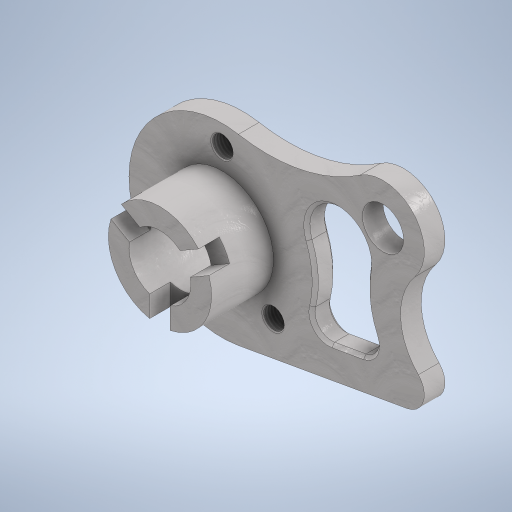
# Autodesk Inventor part: Curved Disc new
Saved by Autodesk Inventor 2023 (Build 270158030, 158C)
## iProperties
Created: 2020-06-23
Part Number: Curved Disc new
Material: Steel, Mild, Welded
Document SubType Name: Modeling
Designer: Smit Ambardekar
Density: 7.85 g/cm^3
Appearance: Weld - Steel Mild
Author: Smit Ambardekar
Autodesk Inventor part; units mm, degrees
ref_plane "YZ Plane" through (0, 0, 0) normal (1, 0, 0) x (0, 1, 0)
ref_plane "XZ Plane" through (0, 0, 0) normal (0, 1, 0) x (-1, 0, 0)
ref_plane "XY Plane" through (0, 0, 0) normal (0, 0, 1) x (1, 0, 0)
sketch "Sketch1" plane through (0, 0, 0) normal (0, 0, 1) x (1, 0, 0)
  arc A0 (8.0041, 44.2824) -> (7.8263, -44.3142) centre (0, 0) ccw
  arc A1 (8.0041, 44.2824) -> (66.8467, 56.6014) centre (22.2337, 123.0068) ccw
  arc A2 (93.3944, 27.2324) -> (66.8467, 56.6014) centre (78, 40) ccw
  arc A3 (89.7392, -29.8476) -> (95.1215, -12.9797) centre (88, -20) ccw
  arc A4 (93.3944, 27.2324) -> (95.1215, -12.9797) centre (116.4861, 8.081) ccw
  line L0 (7.8263, -44.3142) -> (89.7392, -29.8476)
  circle A5 centre (78, 40) radius 10
  arc A6 (70.8456, 19.3234) -> (42.1311, 16.5) centre (56.0864, 22) ccw
  arc A7 (43.9366, -10.8099) -> (53.0508, -21.095) centre (51.5602, -13.2351) ccw
  line L1 (53.0508, -21.095) -> (68.3146, -18.3992)
  arc A8 (68.3146, -18.3992) -> (74.1186, -7.243) centre (66.8289, -10.5384) ccw
  arc A9 (70.8456, 19.3234) -> (74.1186, -7.243) centre (115.1234, 11.2936) ccw
  arc A10 (8.0041, 44.2824) -> (7.8263, -44.3142) centre (0, 0) ccw
  arc A11 (43.9366, -10.8099) -> (42.1311, 16.5) centre (0, 0) ccw
  circle A12 centre (0, 35) radius 5
  line L2 (0, 0) -> (35, 0) construction
  circle A13 centre (-24.7487, -24.7487) radius 5
  circle A14 centre (24.7487, -24.7487) radius 5
  dimension "d1" = 160
  dimension "d2" = 40
  dimension "d3" = 40
  dimension "d4" = 78
  dimension "d6" = 20
  dimension "d7" = 88
  dimension "d8" = 20
  dimension "d9" = 60
  dimension "d10" = 20
  dimension "d12" = 30
  dimension "d13" = 22
  dimension "d22" = 16
  dimension "d23" = 15.5
  dimension "d26" = 90
  dimension "d29" = 10
  dimension "d32" = 10
  dimension "d33" = 10
  dimension "d76" = 15
  constraints: 22 point on circle, 15 centre point, 8 tangent, 6 end point, 4 coincident, 1 horizontal, 1 parallel
  measures "d1" diameter of A1
  measures "d2" diameter of A2
  measures "d3" vertical distance of point (0, 0) A2.centre
  measures "d4" horizontal distance of A2.centre point (0, 0)
  measures "d6" diameter of A3
  measures "d7" horizontal distance of point (0, 0) A3.centre
  measures "d8" vertical distance of A3.centre point (0, 0)
  measures "d9" diameter of A4
  measures "d10" diameter of A5
  measures "d12" diameter of A6
  measures "d13" vertical distance of point (0, 0) A6.centre
  measures "d22" diameter of A7
  measures "d23" distance of L1.end L1.start
  measures "d26" diameter of A9
  measures "d29" diameter of A12
  measures "d32" diameter of A13
  measures "d33" diameter of A14
  measures "d76" distance between parallel lines of L0 L1
extrude "Extrusion1" add sketch "Sketch1" along normal blind 10
sketch "Sketch2" plane through (0, 0, 10) normal (0, 0, 1) x (1, 0, 0)
  circle A0 centre (0, 0) radius 25
  circle A1 centre (0, 0) radius 15
  line L0 (0, 0) -> (25, 0) construction
  line L1 (0, 0) -> (25, 0) construction
  line L2 (-5, -15) -> (-5, -24.4949)
  line L3 (5, -24.4949) -> (5, -15)
  line L4 (-5, -15) -> (-5, -14.1421)
  line L5 (5, -15) -> (5, -14.1421)
  line L6 (0, 0) -> (30, 0) construction
  line L7 (0, 0) -> (30, 0) construction
  line L8 (-23.7132, 7.9173) -> (-14.7474, 2.7409)
  line L9 (-9.7474, 11.4012) -> (-18.7132, 16.5776)
  line L10 (18.7132, 16.5776) -> (9.7474, 11.4012)
  line L11 (14.7474, 2.7409) -> (23.7132, 7.9173)
  dimension "d36" = 50
  dimension "d37" = 30
  dimension "d59" = 10
  constraints: 24 end point, 11 point on circle, 4 horizontal, 3 parallel, 2 centre point, 2 coincident, 2 vertical
  measures "d36" diameter of A0
  measures "d37" diameter of A1
  measures "d59" distance of L11.end L10.start
extrude "Extrusion2" add sketch "Sketch2" along normal blind 30 contours A0 L3 L5 A1 L11 | L10 A1 L9 A0 | A0 L8 A1 L4 L2
chamfer "Chamfer1" distance 0.5 angle 45 6 edges at (-29.7487, -24.7487, 10) (-5, 35, 10) (19.7487, -24.7487, 0) (19.7487, -24.7487, 10) (-29.7487, -24.7487, 0) (-5, 35, 0)
chamfer "Chamfer2" distance 1.5 angle 45 6 edges at (45.5728, -18.5409, 0) (45.1483, 2.9848, 0) (54.6186, 36.928, 0) (70.4611, 5.7912, 0) (73.9259, -14.2306, 0) (60.6827, -19.7471, 0)
sketch "Sketch3" plane through (0, 0, 10) normal (0, 0, 1) x (1, 0, 0)
  line L0 (23.7132, 7.9173) -> (14.7474, 2.7409) projected
  circle A0 centre (0, 0) radius 25
  circle A1 centre (0, 0) radius 15
  line L1 (9.7474, 11.4012) -> (18.7132, 16.5776) projected
  line L2 (9.7474, 11.4012) -> (18.7132, 16.5776)
  line L3 (14.7474, 2.7409) -> (23.7132, 7.9173)
  line L4 (5, -14.1421) -> (5, -24.4949)
  line L5 (-5, -24.4949) -> (-5, -14.1421) projected
  line L6 (-5, -14.1421) -> (-5, -24.4949)
  line L7 (-14.7474, 2.7409) -> (-23.7132, 7.9173) projected
  line L8 (-23.7132, 7.9173) -> (-14.7474, 2.7409)
  line L9 (-18.7132, 16.5776) -> (-9.7474, 11.4012) projected
  line L10 (-18.7132, 16.5776) -> (-9.7474, 11.4012)
  constraints: 12 end point, 4 collinear, 2 centre point, 2 coincident, 2 point on circle, 1 vertical
extrude "Extrusion3" add sketch "Sketch3" along normal blind 20 contours L0 A1 L1 A0 | A0 L5 A1 L4 | L9 A1 L7 A0
sketch "Sketch4" plane through (0, 0, 10) normal (0, 0, 1) x (1, 0, 0)
  circle A0 centre (0, 0) radius 15
  constraints: 1 centre point, 1 coincident
extrude "Extrusion4" cut sketch "Sketch4" against normal blind 10
thread "Thread1" size "M10x1.5" class "6H" standard "ANSI Metric M Profile" length 23.2
thread "Thread2" size "M10x1.5" class "6H" standard "ANSI Metric M Profile" length 23.2
thread "Thread3" size "M10x1.5" class "6H" standard "ANSI Metric M Profile" length 23.2
chamfer "Chamfer4" distance 1.5 angle 45 6 edges at (54.6186, 36.928, 10) (70.4611, 5.7912, 10) (73.9259, -14.2306, 10) (45.1483, 2.9848, 10) (45.5728, -18.5409, 10) (60.6827, -19.7471, 10)
body "Solid1"
